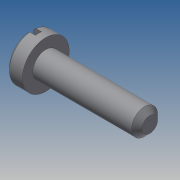
# Autodesk Inventor part: Schlitzschrauebe_ra8846s
Saved by Autodesk Inventor 2021 (Build 250183000, 183)
## iProperties
Created: 2020-11-16
Part Number: Schlitzschrauebe_ra8846s
Material: Allgemein
Document SubType Name: Modeling
Designer: Sander
Density: 1 g/cm^3
Appearance: Vorgabe
Author: Sander
Autodesk Inventor part; units mm, degrees
ref_plane "YZ-Ebene" through (0, 0, 0) normal (1, 0, 0) x (0, 1, 0)
ref_plane "XZ-Ebene" through (0, 0, 0) normal (0, 1, 0) x (-1, 0, 0)
ref_plane "XY-Ebene" through (0, 0, 0) normal (0, 0, 1) x (1, 0, 0)
sketch "Skizze1" plane through (0, 0, 0) normal (0, 0, 1) x (1, 0, 0)
  line L0 (-2.3, 0) -> (13.8, 0) projected
  line L1 (0, -0.4499) -> (0, 2.6994) projected
  line L2 (0, 2.2495) -> (1.5, 2.2495)
  line L3 (1.5, 2.2495) -> (1.5, 1.2495)
  line L4 (1.5, 1.2495) -> (11.5, 1.25)
  line L5 (11.5, 1.25) -> (11.5, 0)
  point P0 (0, 0)
  dimension "d0" = 1.5
  dimension "d1" = 1
  dimension "d2" = 10
  dimension "d3" = 1.25
  constraints: 8 end point, 2 point on line
  measures "d0" distance of L2.start L2.end
  measures "d1" distance of L2.end L3.end
  measures "d2" distance of L3.end L4.end
  measures "d3" distance of L4.end L5.end
revolve "Umdrehung1" add sketch "Skizze1" angle 360 about axis through (-10, 0, 0) along (1, 0, 0)
sketch "Skizze2" plane through (0, 0, 0) normal (-1, 0, 0) x (0, 0, 1)
  circle A0 centre (0, 0) radius 2.2495 projected
  line L0 (-3.1493, 0) -> (3.1493, 0) projected
  line L1 (2.2294, 0.3) -> (-2.2294, 0.3)
  line L2 (2.2294, -0.3) -> (-2.2294, -0.3)
  dimension "d6" = 0.6
  constraints: 4 end point, 4 point on circle, 2 parallel, 1 horizontal, 1 other
  measures "d6" distance between parallel lines of L2 L1
extrude "Extrusion1" cut sketch "Skizze2" against normal blind 0.8 contours L0 A0 L1 | A0 L2 L0
chamfer "Fase1" distance 0.25 angle 45 3 edges at (0, 1.6934, 1.4808) (0, 1.6934, -1.4808) (0, -2.2495, 0)
chamfer "Fase2" distance 0.5 angle 45 1 edges at (11.5, -1.25, 0)
